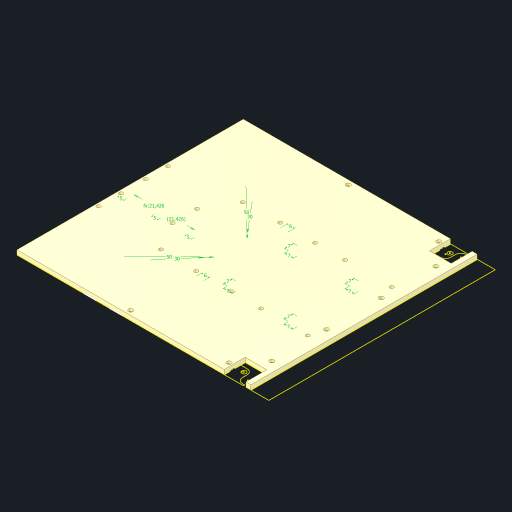
# Autodesk Inventor part: base
Saved by Autodesk Inventor 2023 (Build 270158000, 158)
## iProperties
Created: 2024-05-25
Part Number: base
Material: Nylon 6
Document SubType Name: Modeling
Designer: szymo
Density: 1.12 g/cm^3
Appearance: Nylon 6
Mass: 126.189 g
Surface Area: 671.47 cm^2
Volume: 112.669 cm^3
Author: szymo
Autodesk Inventor part; units mm, degrees
ref_plane "YZ Plane" through (0, 0, 0) normal (1, 0, 0) x (0, 1, 0)
ref_plane "XZ Plane" through (0, 0, 0) normal (0, 1, 0) x (-1, 0, 0)
ref_plane "XY Plane" through (0, 0, 0) normal (0, 0, 1) x (1, 0, 0)
sketch "Sketch1" plane through (0, 0, 0) normal (0, 1, 0) x (-1, 0, 0)
  line L0 (99, 89) -> (-99, 89)
  line L1 (-99, 89) -> (-99, -89)
  line L2 (-99, -89) -> (99, -89)
  line L3 (99, -89) -> (99, 89)
  line L4 (99, 89) -> (-99, -89) construction
  line L5 (-99, 89) -> (99, -89) construction
  line L6 (-85, 89) -> (-85, -89)
  line L7 (-64, 89) -> (-64, 72.5)
  line L8 (-64, 72.5) -> (-81, 72.5)
  line L9 (-81, -72.5) -> (-64, -72.5)
  line L10 (-64, -72.5) -> (-64, -89)
  line L11 (-81, -89) -> (-81, 89)
  point P0 (0, 0)
  dimension "d0" = 198
  dimension "d1" = 178
  dimension "d2" = 14
  dimension "d3" = 16.5
  dimension "d4" = 16.5
  dimension "d9" = 4
  dimension "d10" = 17
  dimension "d11" = 17
  constraints: 24 end point, 8 point on line, 6 perpendicular, 2 horizontal, 2 midpoint, 2 parallel, 1 vertical
  measures "d0" distance of L2.end L1.end
  measures "d1" distance of L1.end L0.end
  measures "d2" distance between parallel lines of L6 L1
  measures "d3" distance between parallel lines of L0 L8
  measures "d4" distance between parallel lines of L9 L2
  measures "d9" distance between parallel lines of L11 L6
  measures "d10" distance between parallel lines of L10 L11
  measures "d11" distance between parallel lines of L11 L7
extrude "Extrusion1" add sketch "Sketch1" along normal blind 3.5 contours L3 L2 L10 L9 L11 L8 L7 L0 | L11 L2 L6 L0
sketch "Sketch2" plane through (0, 0, 0) normal (0, -1, 0) x (1, 0, 0)
  circle A0 centre (-13, -85.5) radius 2.25 projected
  circle A1 centre (61.25, -82.5) radius 2.25 projected
  circle A2 centre (77, -64.5) radius 1.2295 projected
  circle A3 centre (77, -21.5) radius 1.2295 projected
  circle A4 centre (77, 21.5) radius 1.2295 projected
  circle A5 centre (77, 64.5) radius 1.2295 projected
  circle A6 centre (61.25, 82.5) radius 2.25 projected
  circle A7 centre (-13, 85.5) radius 2.25 projected
  point P0 (0, 0)
  constraints: 8 coincident
hole "m3" at (-13, 0, -85.5) at (61.25, 0, -82.5) at (-13, 0, 85.5) at (61.25, 0, 82.5) at (77, 0, 64.5) at (77, 0, 21.5) at (77, 0, -21.5) at (77, 0, -64.5) direction (0, 1, 0) diameter 3.6 end through all countersink diameter 6.7 countersink angle 90 clearance for "Countersunk Flat Head Screw ISO 2009/7046" size "M3" standard "ISO"
sketch "Sketch3" plane through (0, 0, 0) normal (0, -1, 0) x (1, 0, 0)
  circle A0 centre (-96.5, -27.3) radius 1.75
  circle A1 centre (-96.5, -9.7) radius 1.75
  circle A2 centre (-96.5, 9.7) radius 1.75
  circle A3 centre (-96.5, 27.3) radius 1.75
  circle A4 centre (-56, 9.7) radius 1.75
  circle A5 centre (-56, -9.7) radius 1.75
  circle A6 centre (-42.5596, -32.1689) radius 1.5
  circle A7 centre (-42.5596, 32.1689) radius 1.75
  circle A8 centre (-13.9698, 33) radius 1.75
  circle A9 centre (13.5198, 33) radius 1.75
  circle A10 centre (37.0073, 33) radius 1.75
  circle A11 centre (73.7355, 33) radius 1.75
  circle A12 centre (73.7355, -33) radius 1.75
  circle A13 centre (37.0073, -33) radius 1.75
  circle A14 centre (-96.5, -27.3) radius 1.75
  circle A15 centre (73.7355, -33) radius 1.75
  circle A16 centre (13.5198, -33) radius 1.75
  circle A17 centre (-42.5596, -32.1689) radius 1.75
  circle A18 centre (-13.9698, -33) radius 1.75
  arc A19 (-94, -25.8) -> (-95, -24.8) centre (-95, -25.8) ccw
  line L0 (-95, -24.8) -> (-99, -24.8)
  line L1 (-99, -29.8) -> (-99, -24.8)
  line L2 (-48.6566, -29.8) -> (-99, -29.8)
  arc A20 (-47.7313, -30.4207) -> (-48.6566, -29.8) centre (-48.6566, -30.8) ccw
  arc A21 (-46.5, -35.5) -> (-47.7313, -30.4207) centre (-63.78, -37) ccw
  line L3 (79, -35.5) -> (-46.5, -35.5)
  line L4 (79, -35.5) -> (79, -30.5)
  line L5 (79, -30.5) -> (-33.3917, -30.5)
  arc A22 (-40.5373, -26.8) -> (-33.3917, -30.5) centre (-33.3917, -21.75) ccw
  line L6 (-40.5373, -26.8) -> (-41.9987, -26.8)
  spline S0 degree 3 poles (-46.8237, -26.8) (-46.5789, -26.8) (-46.2862, -26.7761) (-45.5332, -26.6913) (-44.9243, -26.6) (-44.4112, -26.6) (-43.8981, -26.6) (-43.2892, -26.6913) (-42.5362, -26.7761) (-42.2435, -26.8) (-41.9987, -26.8) knots 0 0 0 0 0.161475 0.161475 0.5 0.5 0.5 0.838525 0.838525 1 1 1 1
  line L7 (-46.8237, -26.8) -> (-94, -26.8)
  line L8 (-94, -26.8) -> (-94, -25.8)
  line L9 (28.681, 30.5) -> (45.3337, 30.5)
  circle A23 centre (37.0073, 33) radius 1.75
  circle A24 centre (-96.5, 27.3) radius 1.75
  circle A25 centre (73.7355, 33) radius 1.75
  circle A26 centre (13.5198, 33) radius 1.75
  circle A27 centre (-42.5596, 32.1689) radius 1.75
  circle A28 centre (-13.9698, 33) radius 1.75
  arc A29 (-95, 24.8) -> (-94, 25.8) centre (-95, 25.8) ccw
  line L10 (-94, 26.8) -> (-94, 25.8)
  line L11 (-46.8237, 26.8) -> (-94, 26.8)
  spline S1 degree 3 poles (-46.8237, 26.8) (-46.5789, 26.8) (-46.2862, 26.7761) (-45.5332, 26.6913) (-44.9243, 26.6) (-44.4112, 26.6) (-43.8981, 26.6) (-43.2892, 26.6913) (-42.5362, 26.7761) (-42.2435, 26.8) (-41.9987, 26.8) knots 0 0 0 0 0.161475 0.161475 0.5 0.5 0.5 0.838525 0.838525 1 1 1 1
  line L12 (-40.5373, 26.8) -> (-41.9987, 26.8)
  arc A30 (-33.3917, 30.5) -> (-40.5373, 26.8) centre (-33.3917, 21.75) ccw
  line L13 (79, 30.5) -> (-33.3917, 30.5)
  line L14 (79, 35.5) -> (79, 30.5)
  line L15 (79, 35.5) -> (-46.5, 35.5)
  arc A31 (-47.7313, 30.4207) -> (-46.5, 35.5) centre (-63.78, 37) ccw
  arc A32 (-48.6566, 29.8) -> (-47.7313, 30.4207) centre (-48.6566, 30.8) ccw
  line L16 (-48.6566, 29.8) -> (-99, 29.8)
  line L17 (-99, 29.8) -> (-99, 24.8)
  line L18 (-95, 24.8) -> (-99, 24.8)
  point P0 (0, 0)
  constraints: 16 coincident
hole "m2.5" at (73.7355, 0, -33) at (37.0073, 0, -33) at (13.5198, 0, -33) at (-13.9698, 0, -33) at (-42.5596, 0, -32.1689) at (73.7355, 0, 33) at (37.0073, 0, 33) at (13.5198, 0, 33) at (-13.9698, 0, 33) at (-42.5596, 0, 32.1689) at (-56, 0, 9.7) at (-56, 0, -9.7) at (-96.5, 0, -9.7) at (-96.5, 0, 9.7) at (-96.5, 0, 27.3) at (-96.5, 0, -27.3) direction (0, 1, 0) diameter 3.1 end through all countersink diameter 5.8 countersink angle 90 clearance for "Countersunk Flat Head Screw ISO 2009/7046" size "M2.5" standard "ISO"
sketch "Sketch4" plane through (0, 0, 0) normal (0, 1, 0) x (1, 0, 0)
  line L0 (-36.8852, -40.5) -> (-31.5, -40.5)
  line L1 (-31.5, -40.5) -> (-26.1148, -40.5)
  line L2 (-26.1148, -40.5) -> (-26.1148, -68.2)
  line L3 (-26.1148, -68.2) -> (-36.8852, -68.2)
  line L4 (-36.8852, -68.2) -> (-36.8852, -40.5)
  line L5 (-26.1148, 40.5) -> (-31.5, 40.5)
  line L6 (-31.5, 40.5) -> (-36.8852, 40.5)
  line L7 (-36.8852, 40.5) -> (-36.8852, 68.2)
  line L8 (-36.8852, 68.2) -> (-26.1148, 68.2)
  line L9 (-26.1148, 68.2) -> (-26.1148, 40.5)
  circle A0 centre (70, 82.5) radius 1.75
  circle A1 centre (61.25, 82.5) radius 2.25
  circle A2 centre (-13, 85.5) radius 2.25
  line L10 (58, 86) -> (-6.5359, 86)
  arc A3 (-6.5359, 86) -> (-10.018, 83.9686) centre (-6.5359, 82) ccw
  arc A4 (-13, 81.9686) -> (-10.018, 83.9686) centre (-13.5, 85.9373) ccw
  arc A5 (-13, 81.9686) -> (-16.5, 78) centre (-12.5, 78) ccw
  line L11 (-16.5, 78) -> (-16.5, 74)
  line L12 (-16.5, 74) -> (-24.275, 74)
  line L13 (-24.275, 74) -> (-24.275, 88)
  line L14 (-24.275, 88) -> (-38.725, 88)
  line L15 (-38.725, 88) -> (-38.725, 74)
  line L16 (-38.725, 74) -> (-46.5, 74)
  line L17 (-46.5, 89) -> (-46.5, 74)
  line L18 (-46.5, 89) -> (79, 89)
  line L19 (79, 89) -> (79, 88)
  line L20 (79, 88) -> (77.25, 88)
  arc A6 (77.25, 88) -> (73, 83.75) centre (77.25, 83.75) ccw
  line L21 (73, 83.75) -> (73, 80)
  arc A7 (69, 76) -> (73, 80) centre (69, 80) ccw
  line L22 (69, 76) -> (62, 76)
  arc A8 (58, 80) -> (62, 76) centre (62, 80) ccw
  line L23 (58, 86) -> (58, 80)
  circle A9 centre (61.25, -82.5) radius 2.25
  circle A10 centre (-13, -85.5) radius 2.25
  line L24 (58, -86) -> (-6.5359, -86)
  line L25 (58, -86) -> (58, -80)
  arc A11 (62, -76) -> (58, -80) centre (62, -80) ccw
  line L26 (69, -76) -> (62, -76)
  arc A12 (73, -80) -> (69, -76) centre (69, -80) ccw
  line L27 (73, -83.75) -> (73, -80)
  arc A13 (73, -83.75) -> (77.25, -88) centre (77.25, -83.75) ccw
  line L28 (79, -88) -> (77.25, -88)
  line L29 (79, -89) -> (79, -88)
  line L30 (-46.5, -89) -> (79, -89)
  line L31 (-46.5, -89) -> (-46.5, -74)
  line L32 (-38.725, -74) -> (-46.5, -74)
  line L33 (-38.725, -88) -> (-38.725, -74)
  line L34 (-24.275, -88) -> (-38.725, -88)
  line L35 (-24.275, -74) -> (-24.275, -88)
  line L36 (-16.5, -74) -> (-24.275, -74)
  line L37 (-16.5, -78) -> (-16.5, -74)
  arc A14 (-16.5, -78) -> (-13, -81.9686) centre (-12.5, -78) ccw
  arc A15 (-10.018, -83.9686) -> (-13, -81.9686) centre (-13.5, -85.9373) ccw
  arc A16 (-10.018, -83.9686) -> (-6.5359, -86) centre (-6.5359, -82) ccw
  circle A17 centre (70, -79.5) radius 1.75
  circle A18 centre (37.0073, 33) radius 1.75
  circle A19 centre (-96.5, 27.3) radius 1.75
  circle A20 centre (73.7355, 33) radius 1.75
  circle A21 centre (13.5198, 33) radius 1.75
  circle A22 centre (-42.5596, 32.1689) radius 1.75
  circle A23 centre (-13.9698, 33) radius 1.75
  arc A24 (-95, 24.8) -> (-94, 25.8) centre (-95, 25.8) ccw
  line L38 (-95, 24.8) -> (-99, 24.8)
  line L39 (-99, 29.8) -> (-99, 24.8)
  line L40 (-48.6566, 29.8) -> (-99, 29.8)
  arc A25 (-48.6566, 29.8) -> (-47.7313, 30.4207) centre (-48.6566, 30.8) ccw
  arc A26 (-47.7313, 30.4207) -> (-46.5, 35.5) centre (-63.78, 37) ccw
  line L41 (79, 35.5) -> (-46.5, 35.5)
  line L42 (79, 35.5) -> (79, 30.5)
  line L43 (79, 30.5) -> (-33.3917, 30.5)
  arc A27 (-33.3917, 30.5) -> (-40.5373, 26.8) centre (-33.3917, 21.75) ccw
  line L44 (-40.5373, 26.8) -> (-41.9987, 26.8)
  spline S0 degree 3 poles (-46.8237, 26.8) (-46.5789, 26.8) (-46.2862, 26.7761) (-45.5332, 26.6913) (-44.9243, 26.6) (-44.4112, 26.6) (-43.8981, 26.6) (-43.2892, 26.6913) (-42.5362, 26.7761) (-42.2435, 26.8) (-41.9987, 26.8) knots 0 0 0 0 0.161475 0.161475 0.5 0.5 0.5 0.838525 0.838525 1 1 1 1
  line L45 (-46.8237, 26.8) -> (-94, 26.8)
  line L46 (-94, 26.8) -> (-94, 25.8)
  circle A28 centre (37.0073, -33) radius 1.75
  circle A29 centre (-96.5, -27.3) radius 1.75
  circle A30 centre (73.7355, -33) radius 1.75
  circle A31 centre (13.5198, -33) radius 1.75
  circle A32 centre (-42.5596, -32.1689) radius 1.75
  circle A33 centre (-13.9698, -33) radius 1.75
  arc A34 (-94, -25.8) -> (-95, -24.8) centre (-95, -25.8) ccw
  line L47 (-94, -26.8) -> (-94, -25.8)
  line L48 (-46.8237, -26.8) -> (-94, -26.8)
  spline S1 degree 3 poles (-46.8237, -26.8) (-46.5789, -26.8) (-46.2862, -26.7761) (-45.5332, -26.6913) (-44.9243, -26.6) (-44.4112, -26.6) (-43.8981, -26.6) (-43.2892, -26.6913) (-42.5362, -26.7761) (-42.2435, -26.8) (-41.9987, -26.8) knots 0 0 0 0 0.161475 0.161475 0.5 0.5 0.5 0.838525 0.838525 1 1 1 1
  line L49 (-40.5373, -26.8) -> (-41.9987, -26.8)
  arc A35 (-40.5373, -26.8) -> (-33.3917, -30.5) centre (-33.3917, -21.75) ccw
  line L50 (79, -30.5) -> (-33.3917, -30.5)
  line L51 (79, -35.5) -> (79, -30.5)
  line L52 (79, -35.5) -> (-46.5, -35.5)
  arc A36 (-46.5, -35.5) -> (-47.7313, -30.4207) centre (-63.78, -37) ccw
  arc A37 (-47.7313, -30.4207) -> (-48.6566, -29.8) centre (-48.6566, -30.8) ccw
  line L53 (-48.6566, -29.8) -> (-99, -29.8)
  line L54 (-99, -29.8) -> (-99, -24.8)
  line L55 (-95, -24.8) -> (-99, -24.8)
  line L56 (44.7969, 39.7458) -> (-15.2031, 39.7458) construction
  line L57 (-15.2031, 39.7458) -> (-15.2031, 69.7458) construction
  line L58 (44.7969, 69.7458) -> (-15.2031, 69.7458) construction
  line L59 (44.7969, 39.7458) -> (44.7969, 69.7458) construction
  line L60 (44.5627, -68.989) -> (-15.4373, -68.989) construction
  line L61 (-15.4373, -68.989) -> (-15.4373, -38.989) construction
  line L62 (44.5627, -38.989) -> (-15.4373, -38.989) construction
  line L63 (44.5627, -68.989) -> (44.5627, -38.989) construction
  line L64 (85, 89) -> (99, 89)
  line L65 (99, 89) -> (99, -89)
  line L66 (85, -89) -> (99, -89)
  line L67 (85, 89) -> (85, -89)
  circle A38 centre (77, -21.5) radius 1.2295
  circle A39 centre (77, 64.5) radius 1.2295
  circle A40 centre (77, 21.5) radius 1.2295
  circle A41 centre (77, -64.5) radius 1.2295
  line L68 (70, 72) -> (79, 72)
  arc A42 (79, 72) -> (81, 74) centre (79, 74) ccw
  line L69 (81, 74) -> (81, 89)
  line L70 (81, 89) -> (85, 89)
  line L71 (85, 89) -> (85, -89)
  line L72 (81, -89) -> (85, -89)
  line L73 (81, -89) -> (81, -74)
  arc A43 (81, -74) -> (79, -72) centre (79, -74) ccw
  line L74 (79, -72) -> (70, -72)
  line L75 (70, -57) -> (70, -72)
  line L76 (70, -57) -> (79, -57)
  arc A44 (79, -57) -> (81, -55) centre (79, -55) ccw
  line L77 (81, -55) -> (81, -31)
  arc A45 (81, -31) -> (79, -29) centre (79, -31) ccw
  line L78 (79, -29) -> (70, -29)
  line L79 (70, -14) -> (70, -29)
  line L80 (70, -14) -> (79, -14)
  arc A46 (79, -14) -> (81, -12) centre (79, -12) ccw
  line L81 (81, -12) -> (81, 12)
  arc A47 (81, 12) -> (79, 14) centre (79, 12) ccw
  line L82 (79, 14) -> (70, 14)
  line L83 (70, 29) -> (70, 14)
  line L84 (70, 29) -> (79, 29)
  arc A48 (79, 29) -> (81, 31) centre (79, 31) ccw
  line L85 (81, 31) -> (81, 55)
  arc A49 (81, 55) -> (79, 57) centre (79, 55) ccw
  line L86 (79, 57) -> (70, 57)
  line L87 (70, 72) -> (70, 57)
  line L88 (60, -27.5) -> (5, -27.5)
  line L89 (5, -27.5) -> (5, 27.5)
  line L90 (5, 27.5) -> (60, 27.5)
  line L91 (60, 27.5) -> (60, -27.5)
  circle A50 centre (56.6, -24.1) radius 1.6
  circle A51 centre (8.4, -24.1) radius 1.6
  circle A52 centre (56.6, 24.1) radius 1.6
  circle A53 centre (8.4, 24.1) radius 1.6
  line L92 (-99, -7) -> (-37.5, -7) construction
  line L93 (-99, 7) -> (-99, -7) construction
  line L94 (-37.5, 7) -> (-99, 7) construction
  line L95 (-37.5, -7) -> (-37.5, 7) construction
  circle A54 centre (-56, 9.7) radius 1.75
  circle A55 centre (-96.5, 9.7) radius 1.75
  arc A56 (-57.5, 12.2) -> (-58.5, 11.2) centre (-57.5, 11.2) ccw
  line L96 (-57.5, 12.2) -> (-54.5, 12.2)
  arc A57 (-53.5, 11.2) -> (-54.5, 12.2) centre (-54.5, 11.2) ccw
  line L97 (-53.5, 11.2) -> (-53.5, 10.2)
  line L98 (-53.5, 10.2) -> (-46.8237, 10.2)
  spline S2 degree 3 poles (-41.9987, 10.2) (-42.2435, 10.2) (-42.5362, 10.2239) (-43.2892, 10.3087) (-43.8981, 10.4) (-44.4112, 10.4) (-44.9243, 10.4) (-45.5332, 10.3087) (-46.2862, 10.2239) (-46.5789, 10.2) (-46.8237, 10.2) knots 0 0 0 0 0.161475 0.161475 0.5 0.5 0.5 0.838525 0.838525 1 1 1 1
  line L99 (-41.9987, 10.2) -> (-41.148, 10.2)
  line L100 (-41.148, 10.2) -> (-41.148, 7.2)
  line L101 (-41.148, 7.2) -> (-99, 7.2)
  line L102 (-99, 7.2) -> (-99, 12.2)
  line L103 (-99, 12.2) -> (-95, 12.2)
  arc A58 (-94, 11.2) -> (-95, 12.2) centre (-95, 11.2) ccw
  line L104 (-94, 10.2) -> (-94, 11.2)
  line L105 (-94, 10.2) -> (-58.5, 10.2)
  line L106 (-58.5, 10.2) -> (-58.5, 11.2)
  circle A59 centre (-56, -9.7) radius 1.75
  circle A60 centre (-96.5, -9.7) radius 1.75
  arc A61 (-58.5, -11.2) -> (-57.5, -12.2) centre (-57.5, -11.2) ccw
  line L107 (-58.5, -10.2) -> (-58.5, -11.2)
  line L108 (-94, -10.2) -> (-58.5, -10.2)
  line L109 (-94, -10.2) -> (-94, -11.2)
  arc A62 (-95, -12.2) -> (-94, -11.2) centre (-95, -11.2) ccw
  line L110 (-99, -12.2) -> (-95, -12.2)
  line L111 (-99, -7.2) -> (-99, -12.2)
  line L112 (-41.148, -7.2) -> (-99, -7.2)
  line L113 (-41.148, -10.2) -> (-41.148, -7.2)
  line L114 (-41.9987, -10.2) -> (-41.148, -10.2)
  spline S3 degree 3 poles (-41.9987, -10.2) (-42.2435, -10.2) (-42.5362, -10.2239) (-43.2892, -10.3087) (-43.8981, -10.4) (-44.4112, -10.4) (-44.9243, -10.4) (-45.5332, -10.3087) (-46.2862, -10.2239) (-46.5789, -10.2) (-46.8237, -10.2) knots 0 0 0 0 0.161475 0.161475 0.5 0.5 0.5 0.838525 0.838525 1 1 1 1
  line L115 (-53.5, -10.2) -> (-46.8237, -10.2)
  line L116 (-53.5, -11.2) -> (-53.5, -10.2)
  arc A63 (-54.5, -12.2) -> (-53.5, -11.2) centre (-54.5, -11.2) ccw
  line L117 (-57.5, -12.2) -> (-54.5, -12.2)
  line L118 (81, 35.5) -> (-46.5, 35.5)
  line L119 (-46.5, 35.5) -> (-46.5, 29.8)
  line L120 (-46.5, 29.8) -> (-99, 29.8)
  line L121 (-99, 29.8) -> (-99, 24.8)
  line L122 (-99, 24.8) -> (-95, 24.8)
  line L123 (-94, 25.8) -> (-94, 26.8)
  line L124 (-94, 26.8) -> (-40.5373, 26.8)
  line L125 (-40.5373, 26.8) -> (70, 26.8)
  line L126 (81, -35.5) -> (-46.5, -35.5)
  line L127 (-46.5, -35.5) -> (-46.5, -29.8)
  line L128 (-46.5, -29.8) -> (-99, -29.8)
  line L129 (-99, -24.8) -> (-99, -29.8)
  line L130 (-99, -24.8) -> (-95, -24.8)
  line L131 (-94, -25.8) -> (-94, -26.8)
  line L132 (-94, -26.8) -> (-40.5373, -26.8)
  line L133 (-40.5373, -26.8) -> (70, -26.8)
  line L134 (60.1, 27.6) -> (53.1, 27.6)
  line L135 (53.1, 27.6) -> (53.1, 20.6)
  line L136 (53.1, 20.6) -> (60.1, 20.6)
  line L137 (60.1, 20.6) -> (60.1, 27.6)
  line L138 (60.1, 27.6) -> (53.1, 20.6) construction
  line L139 (53.1, 27.6) -> (60.1, 20.6) construction
  line L140 (60.1, -20.6) -> (53.1, -20.6)
  line L141 (53.1, -20.6) -> (53.1, -27.6)
  line L142 (53.1, -27.6) -> (60.1, -27.6)
  line L143 (60.1, -27.6) -> (60.1, -20.6)
  line L144 (60.1, -20.6) -> (53.1, -27.6) construction
  line L145 (53.1, -20.6) -> (60.1, -27.6) construction
  line L146 (11.9, -20.6) -> (4.9, -20.6)
  line L147 (4.9, -20.6) -> (4.9, -27.6)
  line L148 (4.9, -27.6) -> (11.9, -27.6)
  line L149 (11.9, -27.6) -> (11.9, -20.6)
  line L150 (11.9, -20.6) -> (4.9, -27.6) construction
  line L151 (4.9, -20.6) -> (11.9, -27.6) construction
  line L152 (11.9, 27.6) -> (4.9, 27.6)
  line L153 (4.9, 27.6) -> (4.9, 20.6)
  line L154 (4.9, 20.6) -> (11.9, 20.6)
  line L155 (11.9, 20.6) -> (11.9, 27.6)
  line L156 (11.9, 27.6) -> (4.9, 20.6) construction
  line L157 (4.9, 27.6) -> (11.9, 20.6) construction
  line L158 (-99, 7.2) -> (-94, 7.2)
  line L159 (-94, 7.2) -> (-94, -7.2)
  line L160 (-94, -7.2) -> (-99, -7.2)
  line L161 (-99, -7.2) -> (-99, 7.2)
  line L162 (-41.148, 7.2) -> (-46.148, 7.2)
  line L163 (-46.148, 7.2) -> (-46.148, -7.2)
  line L164 (-46.148, -7.2) -> (-41.148, -7.2)
  line L165 (-41.148, -7.2) -> (-41.148, 7.2)
  line L166 (-72.574, 7.2) -> (-67.574, 7.2)
  line L167 (-67.574, 7.2) -> (-67.574, -7.2)
  line L168 (-67.574, -7.2) -> (-72.574, -7.2)
  line L169 (-72.574, -7.2) -> (-72.574, 7.2)
  arc A64 (-41.148, 10.2) -> (-13.9698, 33) centre (-43.1088, 40.1359) ccw
  arc A65 (-13.9698, -33) -> (-41.148, -10.2) centre (-43.1088, -40.1359) ccw
  line L170 (-13.9698, 33) -> (-7.9698, 33)
  line L171 (-13.9698, -33) -> (-7.9698, -33)
  arc A66 (-41.148, 0) -> (-7.9698, 33) centre (-55.7201, 47.8294) ccw
  arc A67 (-7.9698, -33) -> (-41.148, 0) centre (-55.7201, -47.8294) ccw
  line L172 (-36.8852, 35.5) -> (-46.5, 35.5)
  line L173 (-46.5, 35.5) -> (-46.5, 89)
  line L174 (-46.5, 89) -> (-36.8852, 89)
  line L175 (-36.8852, 89) -> (-36.8852, 35.5)
  line L176 (-26.1148, 35.5) -> (-16.5, 35.5)
  line L177 (-16.5, 35.5) -> (-16.5, 89)
  line L178 (-16.5, 89) -> (-26.1148, 89)
  line L179 (-26.1148, 89) -> (-26.1148, 35.5)
  line L180 (-46.5, -35.5) -> (-36.8852, -35.5)
  line L181 (-36.8852, -35.5) -> (-36.8852, -89)
  line L182 (-36.8852, -89) -> (-46.5, -89)
  line L183 (-46.5, -89) -> (-46.5, -35.5)
  line L184 (-26.1148, -89) -> (-16.5, -89)
  line L185 (-16.5, -89) -> (-16.5, -35.5)
  line L186 (-16.5, -35.5) -> (-26.1148, -35.5)
  line L187 (-26.1148, -35.5) -> (-26.1148, -89)
  arc A68 (-99, -28.7697) -> (-99, -25.8303) centre (-96.5, -27.3) ccw
  line L188 (-99, -11.1697) -> (-99, -25.8303)
  arc A69 (-99, -11.1697) -> (-99, -8.2303) centre (-96.5, -9.7) ccw
  line L189 (-99, 8.2303) -> (-99, -8.2303)
  arc A70 (-99, 8.2303) -> (-99, 11.1697) centre (-96.5, 9.7) ccw
  line L190 (-99, 25.8303) -> (-99, 11.1697)
  arc A71 (-99, 25.8303) -> (-99, 28.7697) centre (-96.5, 27.3) ccw
  line L191 (-99, 89) -> (-99, 28.7697)
  line L192 (64, 89) -> (-99, 89)
  line L193 (64, 84.4131) -> (64, 89)
  arc A72 (64, 84.4131) -> (64, 80.5869) centre (61.25, 82.5) ccw
  line L194 (64, 72.5) -> (64, 80.5869)
  line L195 (81, 72.5) -> (64, 72.5)
  line L196 (81, 89) -> (81, 72.5)
  line L197 (85, 89) -> (81, 89)
  line L198 (85, -89) -> (85, 89)
  line L199 (81, -89) -> (85, -89)
  line L200 (81, -72.5) -> (81, -89)
  line L201 (64, -72.5) -> (81, -72.5)
  line L202 (64, -80.5869) -> (64, -72.5)
  arc A73 (64, -80.5869) -> (64, -84.4131) centre (61.25, -82.5) ccw
  line L203 (64, -89) -> (64, -84.4131)
  line L204 (-99, -89) -> (64, -89)
  line L205 (-99, -28.7697) -> (-99, -89)
  circle A74 centre (-56, -9.7) radius 2.9
  circle A75 centre (-13.9698, -33) radius 2.9
  circle A76 centre (37.0073, -33) radius 2.9
  circle A77 centre (-42.5596, 32.1689) radius 2.9
  circle A78 centre (13.5198, 33) radius 2.9
  circle A79 centre (73.7355, 33) radius 2.9
  circle A80 centre (37.0073, 33) radius 2.9
  circle A81 centre (-13.9698, 33) radius 2.9
  circle A82 centre (73.7355, -33) radius 2.9
  circle A83 centre (13.5198, -33) radius 2.9
  circle A84 centre (-42.5596, -32.1689) radius 2.9
  circle A85 centre (-56, 9.7) radius 2.9
  circle A86 centre (77, 64.5) radius 3.35
  circle A87 centre (77, -21.5) radius 3.35
  circle A88 centre (-13, 85.5) radius 3.35
  circle A89 centre (-13, -85.5) radius 3.35
  circle A90 centre (77, -64.5) radius 3.35
  circle A91 centre (77, 21.5) radius 3.35
  point P0 (0, 0)
  dimension "d26" = 7
  dimension "d27" = 7
  dimension "d28" = 7
  dimension "d29" = 7
  dimension "d30" = 7
  dimension "d31" = 7
  dimension "d32" = 7
  dimension "d33" = 7
  dimension "d34" = 5
  dimension "d35" = 5
  dimension "d36" = 5
  dimension "d37" = 21.426
  dimension "d38" = 21.426
  dimension "d39" = 30
  dimension "d40" = 30
  dimension "d41" = 6
  dimension "d42" = 6
  dimension "d43" = 50
  dimension "d44" = 50
  constraints: 160 end point, 22 parallel, 19 horizontal, 18 point on line, 16 perpendicular, 9 collinear, 9 midpoint, 8 point on circle, 5 vertical, 4 centre point, 1 tangent, 10 other
  measures "d26" distance of L136.end L135.end
  measures "d27" distance of L135.end L134.end
  measures "d28" distance of L142.end L141.end
  measures "d29" distance of L141.end L140.end
  measures "d30" distance of L148.end L147.end
  measures "d31" distance of L147.end L146.end
  measures "d32" distance of L154.end L153.end
  measures "d33" distance of L153.end L152.end
  measures "d34" distance of L159.end L160.end
  measures "d35" distance of L164.end L163.end
  measures "d36" distance of L167.end L168.end
  measures "d37" distance between parallel lines of L169 L159
  measures "d38" distance between parallel lines of L163 L167
  measures "d39" radius of A64
  measures "d40" radius of A65
  measures "d41" distance of L170.start L170.end
  measures "d42" distance of L171.start L171.end
  measures "d43" radius of A66
  measures "d44" radius of A67
equation "\"d37\" = d38"
body "Solid1"
